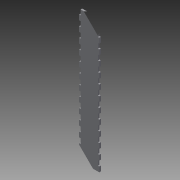
# Autodesk Inventor part: small wall
Saved by Autodesk Inventor 2015 (Build 190159000, 159)
## iProperties
Created: 2015-01-31
Part Number: small wall
Material: Generic
Document SubType Name: Modeling
Designer: Joseph
Density: 1 g/cm^3
Appearance: Default
Author: Joseph
Autodesk Inventor part; units mm, degrees
ref_plane "YZ Plane" through (0, 0, 0) normal (1, 0, 0) x (0, 1, 0)
ref_plane "XZ Plane" through (0, 0, 0) normal (0, 1, 0) x (-1, 0, 0)
ref_plane "XY Plane" through (0, 0, 0) normal (0, 0, 1) x (1, 0, 0)
sketch "Sketch1" plane through (0, 0, 0) normal (0, 0, 1) x (1, 0, 0)
  line L0 (0, 0) -> (0, 20)
  line L1 (79.3918, 0) -> (79.3918, 20) projected
  line L2 (79.3918, 0) -> (0, 0) projected
  line L3 (-0.2277, -520) -> (79.6269, -520) projected
  line L4 (5.4724, 0) -> (74.116, 0)
  line L5 (79.6269, -520) -> (0, -520)
  line L6 (74.116, -20) -> (74.116, 0) projected
  line L7 (74.116, 0) -> (74.116, -20)
  line L8 (74.116, -20) -> (79.5884, -20)
  line L9 (0, -20) -> (5.4724, -20)
  line L10 (5.4724, -20) -> (5.4724, 0)
  line L11 (39.7942, 0) -> (39.7942, -37.2544) construction
  line L12 (0, -20) -> (0, -40)
  line L13 (0, -40) -> (5.4724, -40)
  line L14 (79.5884, -20) -> (79.5884, -40)
  line L15 (79.5884, -40) -> (74.28, -40)
  line L16 (5.4724, -40) -> (5.4724, -60)
  line L17 (5.4724, -60) -> (0, -60)
  line L18 (0, -60) -> (0, -80)
  line L19 (0, -80) -> (5.4724, -80)
  line L20 (5.4724, -80) -> (5.4724, -100)
  line L21 (5.4724, -100) -> (0, -100)
  line L22 (0, -100) -> (0, -120)
  line L23 (0, -120) -> (5.4724, -120)
  line L24 (5.4724, -120) -> (5.4724, -140)
  line L25 (5.4724, -140) -> (0, -140)
  line L26 (0, -140) -> (0, -160)
  line L27 (0, -160) -> (5.4724, -160)
  line L28 (5.4724, -160) -> (5.4724, -180)
  line L29 (5.4724, -180) -> (0, -180)
  line L30 (0, -180) -> (0, -200)
  line L31 (0, -200) -> (5.4724, -200)
  line L32 (5.4724, -200) -> (5.4724, -220)
  line L33 (5.4724, -220) -> (0, -220)
  line L34 (0, -220) -> (0, -240)
  line L35 (0, -240) -> (5.4724, -240)
  line L36 (5.4724, -240) -> (5.4724, -260)
  line L37 (5.4724, -260) -> (0, -260)
  line L38 (0, -260) -> (0, -280)
  line L39 (0, -280) -> (5.4724, -280)
  line L40 (5.4724, -280) -> (5.4724, -300)
  line L41 (5.4724, -300) -> (0, -300)
  line L42 (0, -300) -> (0, -320)
  line L43 (0, -320) -> (5.4724, -320)
  line L44 (5.4724, -320) -> (5.4724, -340)
  line L45 (5.4724, -340) -> (0, -340)
  line L46 (0, -340) -> (0, -360)
  line L47 (0, -360) -> (5.4724, -360)
  line L48 (5.4724, -360) -> (5.4724, -380)
  line L49 (5.4724, -380) -> (0, -380)
  line L50 (0, -380) -> (0, -400)
  line L51 (0, -400) -> (5.4724, -400)
  line L52 (5.4724, -400) -> (5.4724, -420)
  line L53 (5.4724, -420) -> (0, -420)
  line L54 (0, -420) -> (0, -440)
  line L55 (0, -440) -> (5.4724, -440)
  line L56 (5.4724, -440) -> (5.4724, -460)
  line L57 (5.4724, -460) -> (0, -460)
  line L58 (0, -460) -> (0, -480)
  line L59 (0, -480) -> (5.4724, -480)
  line L60 (5.4724, -480) -> (5.4724, -500)
  line L61 (5.4724, -500) -> (0, -500)
  line L62 (0, -500) -> (0, -520)
  line L63 (74.28, -40) -> (74.28, -60)
  line L64 (74.28, -60) -> (79.6269, -60)
  line L65 (79.6269, -60) -> (79.6269, -80)
  line L66 (79.6269, -80) -> (74.28, -80)
  line L67 (74.28, -80) -> (74.28, -100)
  line L68 (74.28, -100) -> (79.6269, -100)
  line L69 (79.6269, -100) -> (79.6269, -120)
  line L70 (79.6269, -120) -> (74.28, -120)
  line L71 (74.28, -120) -> (74.28, -140)
  line L72 (74.28, -140) -> (79.6269, -140)
  line L73 (79.6269, -140) -> (79.6269, -160)
  line L74 (79.6269, -160) -> (74.28, -160)
  line L75 (74.28, -160) -> (74.28, -180)
  line L76 (74.28, -180) -> (79.6269, -180)
  line L77 (79.6269, -180) -> (79.6269, -200)
  line L78 (79.6269, -200) -> (74.28, -200)
  line L79 (74.28, -200) -> (74.28, -220)
  line L80 (74.28, -220) -> (79.6269, -220)
  line L81 (79.6269, -220) -> (79.6269, -240)
  line L82 (79.6269, -240) -> (74.28, -240)
  line L83 (74.28, -240) -> (74.28, -260)
  line L84 (74.28, -260) -> (79.6269, -260)
  line L85 (79.6269, -260) -> (79.6269, -280)
  line L86 (79.6269, -280) -> (74.28, -280)
  line L87 (74.28, -280) -> (74.28, -300)
  line L88 (74.28, -300) -> (79.6269, -300)
  line L89 (79.6269, -300) -> (79.6269, -320)
  line L90 (79.6269, -320) -> (74.28, -320)
  line L91 (74.28, -320) -> (74.28, -340)
  line L92 (74.28, -340) -> (79.6269, -340)
  line L93 (79.6269, -340) -> (79.6269, -360)
  line L94 (79.6269, -360) -> (74.28, -360)
  line L95 (74.28, -360) -> (74.28, -380)
  line L96 (74.28, -380) -> (79.6269, -380)
  line L97 (79.6269, -380) -> (79.6269, -400)
  line L98 (79.6269, -400) -> (74.28, -400)
  line L99 (74.28, -400) -> (74.28, -420)
  line L100 (74.28, -420) -> (79.6269, -420)
  line L101 (79.6269, -420) -> (79.6269, -440)
  line L102 (79.6269, -440) -> (74.28, -440)
  line L103 (74.28, -440) -> (74.28, -460)
  line L104 (74.28, -460) -> (79.6269, -460)
  line L105 (79.6269, -460) -> (79.6269, -480)
  line L106 (79.6269, -480) -> (74.28, -480)
  line L107 (74.28, -480) -> (74.28, -500)
  line L108 (74.28, -500) -> (79.6269, -500)
  line L109 (79.6269, -500) -> (79.6269, -520)
  dimension "d16" = 20
  dimension "d17" = 20
  dimension "d18" = 20
  dimension "d19" = 20
  dimension "d20" = 20
  dimension "d21" = 20
  dimension "d22" = 20
  dimension "d23" = 20
  dimension "d24" = 20
  dimension "d25" = 20
  dimension "d26" = 20
  dimension "d27" = 20
  dimension "d28" = 20
  dimension "d29" = 20
  dimension "d30" = 20
  dimension "d31" = 20
  dimension "d32" = 20
  dimension "d33" = 20
  dimension "d34" = 20
  dimension "d35" = 20
  dimension "d36" = 20
  dimension "d37" = 20
  dimension "d38" = 20
  dimension "d39" = 20
  constraints: 212 end point, 82 point on line, 52 perpendicular, 7 equal length, 7 vertical, 4 parallel, 2 horizontal, 1 collinear, 1 midpoint
  measures "d16" distance of L9.start L12.end
  measures "d17" distance of L13.end L16.end
  measures "d18" distance of L17.end L18.end
  measures "d19" distance of L19.end L20.end
  measures "d20" distance of L21.end L22.end
  measures "d21" distance of L23.end L24.end
  measures "d22" distance of L25.end L26.end
  measures "d23" distance of L27.end L28.end
  measures "d24" distance of L29.end L30.end
  measures "d25" distance of L31.end L32.end
  measures "d26" distance of L35.end L36.end
  measures "d27" distance of L37.end L38.end
  measures "d28" distance of L39.end L40.end
  measures "d29" distance of L41.end L42.end
  measures "d30" distance of L43.end L44.end
  measures "d31" distance of L45.end L46.end
  measures "d32" distance of L47.end L48.end
  measures "d33" distance of L49.end L50.end
  measures "d34" distance of L51.end L52.end
  measures "d35" distance of L53.end L54.end
  measures "d36" distance of L55.end L56.end
  measures "d37" distance of L57.end L58.end
  measures "d38" distance of L59.end L60.end
  measures "d39" distance of L61.end L5.end
extrude "Extrusion1" add sketch "Sketch1" against normal blind 6.35
body "Solid1"
